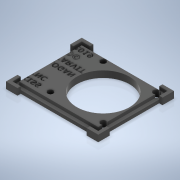
# Autodesk Inventor part: TNC Cover
Saved by Autodesk Inventor 2020.1 (Build 241239000, 239)
## iProperties
Created: 2019-09-18
Part Number: TNC Cover
Material: PC/ABS Plastic
Document SubType Name: Modeling
Designer: Logan
Density: 0.357273 g/cm^3
Appearance: Smooth - Black
Author: Logan
Autodesk Inventor part; units mm, degrees
(part 1 of 2)
ref_plane "YZ Plane" through (0, 0, 0) normal (1, 0, 0) x (0, 1, 0)
ref_plane "XZ Plane" through (0, 0, 0) normal (0, 1, 0) x (-1, 0, 0)
ref_plane "XY Plane" through (0, 0, 0) normal (0, 0, 1) x (1, 0, 0)
sketch "Sketch1" plane through (0, 0, 0) normal (0, 1, 0) x (-1, 0, 0)
  line L0 (0, 0) -> (52, 0)
  line L1 (52, 0) -> (52, -42)
  line L2 (52, -42) -> (0, -42)
  line L3 (0, -42) -> (0, 0)
  line L4 (52, 0) -> (0, 0)
  line L5 (0, 0) -> (0, -2)
  line L6 (0, -2) -> (52, -2)
  line L7 (52, -2) -> (52, 0)
  line L8 (0, 0) -> (2, 0)
  line L9 (2, 0) -> (2, -42)
  line L10 (2, -42) -> (0, -42)
  line L11 (0, -42) -> (0, 0)
  line L12 (52, -42) -> (0, -42)
  line L13 (0, -42) -> (0, -40)
  line L14 (0, -40) -> (52, -40)
  line L15 (52, -40) -> (52, -42)
  line L16 (52, -42) -> (50, -42)
  line L17 (50, -42) -> (50, 0)
  line L18 (50, 0) -> (52, 0)
  line L19 (52, 0) -> (52, -42)
  dimension "d0" = 52
  dimension "d1" = 42
  constraints: 40 end point, 10 parallel, 5 horizontal, 5 perpendicular, 4 point on line
  measures "d0" distance of L1.end L2.end
  measures "d1" distance of L0.end L1.end
extrude "Extrusion1" add sketch "Sketch1" along normal blind 2
sketch "Sketch2" plane through (0, 2, 0) normal (0, 1, 0) x (1, 0, 0)
  line L0 (-52, 42) -> (-52, 0) projected
  line L1 (0, 0) -> (0, 42) projected
  line L2 (-52, 0) -> (0, 0)
  line L3 (0, 0) -> (0, 2)
  line L4 (0, 2) -> (-52, 2)
  line L5 (-52, 2) -> (-52, 0)
  line L6 (0, 42) -> (-52, 42) projected
  line L7 (0, 0) -> (-2, 0)
  line L8 (-2, 0) -> (-2, 42)
  line L9 (-2, 42) -> (0, 42)
  line L10 (0, 42) -> (0, 0)
  line L11 (0, 42) -> (-52, 42)
  line L12 (-52, 42) -> (-52, 40)
  line L13 (-52, 40) -> (0, 40)
  line L14 (0, 40) -> (0, 42)
  line L15 (-52, 0) -> (0, 0) projected
  line L16 (-52, 42) -> (-50, 42)
  line L17 (-50, 42) -> (-50, 0)
  line L18 (-50, 0) -> (-52, 0)
  line L19 (-52, 0) -> (-52, 42)
  line L20 (-2, 2) -> (-50, 2)
  line L21 (-50, 2) -> (-50, 4)
  line L22 (-50, 4) -> (-2, 4)
  line L23 (-2, 4) -> (-2, 2)
  line L24 (-50, 2) -> (-48, 2)
  line L25 (-48, 2) -> (-48, 40)
  line L26 (-48, 40) -> (-50, 40)
  line L27 (-50, 40) -> (-50, 2)
  line L28 (-50, 40) -> (-2, 40)
  line L29 (-2, 40) -> (-2, 38)
  line L30 (-2, 38) -> (-50, 38)
  line L31 (-50, 38) -> (-50, 40)
  line L32 (-2, 40) -> (-4, 40)
  line L33 (-4, 40) -> (-4, 2)
  line L34 (-4, 2) -> (-2, 2)
  line L35 (-2, 2) -> (-2, 40)
  point P0 (-50, 2)
  point P1 (-2, 40)
  constraints: 64 end point, 16 parallel, 10 point on line, 8 horizontal, 8 perpendicular
extrude "Extrusion2" add sketch "Sketch2" along normal blind 2 contours L13 L25 L30 L17 | L17 L22 L25 L4 | L13 L33 L30 L25 | L30 L25 L22 L17 | L8 L30 L33 L13 | L25 L22 L33 L4 | L30 L33 L22 L25 | L8 L22 L33 L30 | L33 L22 L8 L4
sketch "Sketch3" plane through (0, 2, 0) normal (0, 1, 0) x (1, 0, 0)
  line L0 (-52, 0) -> (0, 0) projected
  line L1 (0, 0) -> (2, 0)
  line L2 (2, 0) -> (2, 5)
  line L3 (2, 5) -> (0, 5)
  line L4 (0, 5) -> (0, 0)
  line L5 (0, 0) -> (-5, 0)
  line L6 (-5, 0) -> (-5, -2)
  line L7 (-5, -2) -> (0, -2)
  line L8 (0, -2) -> (0, 0)
  line L9 (0, -2) -> (2, -2)
  line L10 (2, -2) -> (2, 0)
  line L11 (2, 0) -> (0, 0)
  line L12 (0, 0) -> (0, -2)
  line L13 (-52, 0) -> (-47, 0)
  line L14 (-47, 0) -> (-47, -2)
  line L15 (-47, -2) -> (-52, -2)
  line L16 (-52, -2) -> (-52, 0)
  line L17 (-52, -2) -> (-54, -2)
  line L18 (-54, -2) -> (-54, 0)
  line L19 (-54, 0) -> (-52, 0)
  line L20 (-52, 0) -> (-52, -2)
  line L21 (-52, 42) -> (-52, 0) projected
  line L22 (-54, 0) -> (-52, 0)
  line L23 (-52, 0) -> (-52, 5)
  line L24 (-52, 5) -> (-54, 5)
  line L25 (-54, 5) -> (-54, 0)
  line L26 (-52, 42) -> (-54, 42)
  line L27 (-54, 42) -> (-54, 37)
  line L28 (-54, 37) -> (-52, 37)
  line L29 (-52, 37) -> (-52, 42)
  line L30 (-54, 42) -> (-52, 42)
  line L31 (-52, 42) -> (-52, 44)
  line L32 (-52, 44) -> (-54, 44)
  line L33 (-54, 44) -> (-54, 42)
  line L34 (0, 42) -> (-52, 42) projected
  line L35 (-52, 44) -> (-47, 44)
  line L36 (-47, 44) -> (-47, 42)
  line L37 (-47, 42) -> (-52, 42)
  line L38 (-52, 42) -> (-52, 44)
  line L39 (0, 42) -> (-5, 42)
  line L40 (-5, 42) -> (-5, 44)
  line L41 (-5, 44) -> (0, 44)
  line L42 (0, 44) -> (0, 42)
  line L43 (0, 44) -> (2, 44)
  line L44 (2, 44) -> (2, 42)
  line L45 (2, 42) -> (0, 42)
  line L46 (0, 42) -> (0, 44)
  line L47 (0, 42) -> (2, 42)
  line L48 (2, 42) -> (2, 37)
  line L49 (2, 37) -> (0, 37)
  line L50 (0, 37) -> (0, 42)
  dimension "d6" = 5
  constraints: 96 end point, 24 parallel, 13 point on line, 12 horizontal, 12 perpendicular
  measures "d6" distance of L7.end L6.end
extrude "Extrusion3" add sketch "Sketch3" along normal mid plane 4
sketch "Sketch4" plane through (0, 0, 0) normal (0, -1, 0) x (1, 0, 0)
  line L0 (-52, -37) -> (-52, -42) projected
  line L1 (0, -5) -> (0, 0) projected
  line L2 (-52, -42) -> (0, -42)
  line L3 (0, -42) -> (0, 0)
  line L4 (0, 0) -> (-52, 0)
  line L5 (-52, 0) -> (-52, -42)
  line L6 (0, -5) -> (0, -37) projected
  line L7 (-52, -42) -> (0, -42)
  line L8 (0, -42) -> (0, -21)
  line L9 (0, -21) -> (-52, -21)
  line L10 (-52, -21) -> (-52, -42)
  line L11 (-52, -5) -> (-52, 0) projected
  line L12 (0, -21) -> (-52, -21)
  line L13 (-52, -21) -> (-52, 0)
  line L14 (-52, 0) -> (0, 0)
  line L15 (0, 0) -> (0, -21)
  line L16 (-52, -42) -> (-25, -42)
  line L17 (-25, -42) -> (-25, 0)
  line L18 (-25, 0) -> (-52, 0)
  line L19 (-52, 0) -> (-52, -42)
  line L20 (-51.6249, -4.1916) -> (-42.1937, -4.1916) construction
  line L21 (-42.1937, -4.1916) -> (-42.1937, -39.0347) construction
  line L22 (-42.1937, -39.0347) -> (-51.6249, -39.0347) construction
  line L23 (-51.6249, -39.0347) -> (-51.6249, -4.1916) construction
  line L24 (-3, -6) -> (-35, -6)
  line L25 (-35, -6) -> (-35, -38)
  line L26 (-35, -38) -> (-3, -38)
  line L27 (-3, -38) -> (-3, -6)
  circle A0 centre (-3, -6) radius 1.75
  circle A1 centre (-3, -38) radius 1.75
  circle A2 centre (-35, -38) radius 1.75
  circle A3 centre (-35, -6) radius 1.75
  line L28 (-35, -6) -> (-3, -6)
  line L29 (-3, -6) -> (1, -6)
  line L30 (-35, -6) -> (-39, -6)
  line L31 (-35, -6) -> (-35, -2)
  line L32 (-2, -2) -> (-50, -2) projected
  line L33 (-3, -6) -> (-3, -2)
  line L34 (-3, -38) -> (-3, -42)
  line L35 (0, -42) -> (-5, -42) projected
  line L36 (-3, -38) -> (1, -38)
  line L37 (1, -38) -> (-35, -38)
  line L38 (-35, -38) -> (-39, -38)
  line L39 (-39, -38) -> (-35, -38)
  line L40 (-35, -38) -> (-35, -42)
  line L41 (-39, -22) -> (-19, -22)
  circle A4 centre (-19, -22) radius 16
  line L42 (-48.5191, -7.4182) -> (-49.4824, -7.4182)
  line L43 (-49.4824, -7.4182) -> (-50.343, -6.1311)
  line L44 (-50.343, -6.1311) -> (-50.4997, -6.3469)
  line L45 (-50.4997, -6.3469) -> (-50.4997, -7.4182)
  line L46 (-50.4997, -7.4182) -> (-51.2961, -7.4182)
  line L47 (-51.2961, -7.4182) -> (-51.2961, -4.2482)
  line L48 (-51.2961, -4.2482) -> (-50.4997, -4.2482)
  line L49 (-50.4997, -4.2482) -> (-50.4997, -5.6636)
  line L50 (-50.4997, -5.6636) -> (-49.4824, -4.2482)
  line L51 (-49.4824, -4.2482) -> (-48.5654, -4.2482)
  line L52 (-48.5654, -4.2482) -> (-49.6957, -5.7201)
  line L53 (-49.6957, -5.7201) -> (-48.5191, -7.4182)
  line L54 (-46.6824, -7.4182) -> (-48.3881, -7.4182)
  line L55 (-48.3881, -7.4182) -> (-48.3881, -6.8658)
  line L56 (-48.3881, -6.8658) -> (-47.9334, -6.8658)
  line L57 (-47.9334, -6.8658) -> (-47.9334, -4.8005)
  line L58 (-47.9334, -4.8005) -> (-48.3881, -4.8005)
  line L59 (-48.3881, -4.8005) -> (-48.3881, -4.2482)
  line L60 (-48.3881, -4.2482) -> (-46.6824, -4.2482)
  line L61 (-46.6824, -4.2482) -> (-46.6824, -4.8005)
  line L62 (-46.6824, -4.8005) -> (-47.1371, -4.8005)
  line L63 (-47.1371, -4.8005) -> (-47.1371, -6.8658)
  line L64 (-47.1371, -6.8658) -> (-46.6824, -6.8658)
  line L65 (-46.6824, -6.8658) -> (-46.6824, -7.4182)
  spline S0 degree 2 poles (-45.1744, -7.4747) (-45.5392, -7.4747) (-46.089, -7.3334) (-46.3253, -7.2306) knots 0 0 0 1 2 2 2
  line L66 (-46.3253, -7.2306) -> (-46.3253, -6.4754)
  line L67 (-46.3253, -6.4754) -> (-46.2534, -6.4754)
  spline S1 degree 2 poles (-46.2534, -6.4754) (-46.0145, -6.6783) (-45.4416, -6.8967) (-45.1719, -6.8967) knots 0 0 0 1 2 2 2
  spline S2 degree 2 poles (-45.1719, -6.8967) (-45.1025, -6.8967) (-44.879, -6.8658) (-44.8122, -6.835) knots 0 0 0 1 2 2 2
  spline S3 degree 2 poles (-44.8122, -6.835) (-44.73, -6.7991) (-44.6144, -6.668) (-44.6144, -6.5627) knots 0 0 0 1 2 2 2
  spline S4 degree 2 poles (-44.6144, -6.5627) (-44.6144, -6.442) (-44.8019, -6.293) (-44.9304, -6.2596) knots 0 0 0 1 2 2 2
  spline S5 degree 2 poles (-44.9304, -6.2596) (-45.0922, -6.2159) (-45.4596, -6.1414) (-45.6214, -6.0849) knots 0 0 0 1 2 2 2
  spline S6 degree 2 poles (-45.6214, -6.0849) (-45.9888, -5.9565) (-46.3073, -5.5172) (-46.3073, -5.1884) knots 0 0 0 1 2 2 2
  spline S7 degree 2 poles (-46.3073, -5.1884) (-46.3073, -4.744) (-45.5546, -4.1916) (-44.9895, -4.1916) knots 0 0 0 1 2 2 2
  spline S8 degree 2 poles (-44.9895, -4.1916) (-44.7069, -4.1916) (-44.1469, -4.3072) (-43.926, -4.4049) knots 0 0 0 1 2 2 2
  line L68 (-43.926, -4.4049) -> (-43.926, -5.1293)
  line L69 (-43.926, -5.1293) -> (-43.9953, -5.1293)
  spline S9 degree 2 poles (-43.9953, -5.1293) (-44.1726, -4.9777) (-44.6812, -4.7696) (-44.9484, -4.7696) knots 0 0 0 1 2 2 2
  spline S10 degree 2 poles (-44.9484, -4.7696) (-45.0537, -4.7696) (-45.2181, -4.8005) (-45.3106, -4.8416) knots 0 0 0 1 2 2 2
  spline S11 degree 2 poles (-45.3106, -4.8416) (-45.3851, -4.875) (-45.493, -5.0085) (-45.493, -5.0908) knots 0 0 0 1 2 2 2
  spline S12 degree 2 poles (-45.493, -5.0908) (-45.493, -5.2141) (-45.3209, -5.3553) (-45.0742, -5.4119) knots 0 0 0 1 2 2 2
  spline S13 degree 2 poles (-45.0742, -5.4119) (-44.915, -5.4478) (-44.6196, -5.5172) (-44.45, -5.5763) knots 0 0 0 1 2 2 2
  spline S14 degree 2 poles (-44.45, -5.5763) (-44.1212, -5.697) (-43.8001, -6.0978) (-43.8001, -6.4266) knots 0 0 0 1 2 2 2
  spline S15 degree 2 poles (-43.8001, -6.4266) (-43.8001, -6.8992) (-44.5425, -7.4747) (-45.1744, -7.4747) knots 0 0 0 1 2 2 2
  spline S16 degree 2 poles (-42.4129, -7.4747) (-42.7777, -7.4747) (-43.3274, -7.3334) (-43.5637, -7.2306) knots 0 0 0 1 2 2 2
  line L70 (-43.5637, -7.2306) -> (-43.5637, -6.4754)
  line L71 (-43.5637, -6.4754) -> (-43.4918, -6.4754)
  spline S17 degree 2 poles (-43.4918, -6.4754) (-43.2529, -6.6783) (-42.68, -6.8967) (-42.4103, -6.8967) knots 0 0 0 1 2 2 2
  spline S18 degree 2 poles (-42.4103, -6.8967) (-42.341, -6.8967) (-42.1175, -6.8658) (-42.0507, -6.835) knots 0 0 0 1 2 2 2
  spline S19 degree 2 poles (-42.0507, -6.835) (-41.9685, -6.7991) (-41.8529, -6.668) (-41.8529, -6.5627) knots 0 0 0 1 2 2 2
  spline S20 degree 2 poles (-41.8529, -6.5627) (-41.8529, -6.442) (-42.0404, -6.293) (-42.1688, -6.2596) knots 0 0 0 1 2 2 2
  spline S21 degree 2 poles (-42.1688, -6.2596) (-42.3307, -6.2159) (-42.698, -6.1414) (-42.8599, -6.0849) knots 0 0 0 1 2 2 2
  spline S22 degree 2 poles (-42.8599, -6.0849) (-43.2272, -5.9565) (-43.5458, -5.5172) (-43.5458, -5.1884) knots 0 0 0 1 2 2 2
  spline S23 degree 2 poles (-43.5458, -5.1884) (-43.5458, -4.744) (-42.7931, -4.1916) (-42.2279, -4.1916) knots 0 0 0 1 2 2 2
  spline S24 degree 2 poles (-42.2279, -4.1916) (-41.9453, -4.1916) (-41.3853, -4.3072) (-41.1644, -4.4049) knots 0 0 0 1 2 2 2
  line L72 (-41.1644, -4.4049) -> (-41.1644, -5.1293)
  line L73 (-41.1644, -5.1293) -> (-41.2338, -5.1293)
  spline S25 degree 2 poles (-41.2338, -5.1293) (-41.411, -4.9777) (-41.9197, -4.7696) (-42.1868, -4.7696) knots 0 0 0 1 2 2 2
  spline S26 degree 2 poles (-42.1868, -4.7696) (-42.2921, -4.7696) (-42.4566, -4.8005) (-42.549, -4.8416) knots 0 0 0 1 2 2 2
  spline S27 degree 2 poles (-42.549, -4.8416) (-42.6235, -4.875) (-42.7314, -5.0085) (-42.7314, -5.0908) knots 0 0 0 1 2 2 2
  spline S28 degree 2 poles (-42.7314, -5.0908) (-42.7314, -5.2141) (-42.5593, -5.3553) (-42.3127, -5.4119) knots 0 0 0 1 2 2 2
  spline S29 degree 2 poles (-42.3127, -5.4119) (-42.1534, -5.4478) (-41.858, -5.5172) (-41.6885, -5.5763) knots 0 0 0 1 2 2 2
  spline S30 degree 2 poles (-41.6885, -5.5763) (-41.3596, -5.697) (-41.0385, -6.0978) (-41.0385, -6.4266) knots 0 0 0 1 2 2 2
  spline S31 degree 2 poles (-41.0385, -6.4266) (-41.0385, -6.8992) (-41.7809, -7.4747) (-42.4129, -7.4747) knots 0 0 0 1 2 2 2
  line L74 (-50.6873, -12.6375) -> (-50.6873, -10.0712)
  line L75 (-50.6873, -10.0712) -> (-51.6249, -10.0712)
  line L76 (-51.6249, -10.0712) -> (-51.6249, -9.4675)
  line L77 (-51.6249, -9.4675) -> (-48.9533, -9.4675)
  line L78 (-48.9533, -9.4675) -> (-48.9533, -10.0712)
  line L79 (-48.9533, -10.0712) -> (-49.8909, -10.0712)
  line L80 (-49.8909, -10.0712) -> (-49.8909, -12.6375)
  line L81 (-49.8909, -12.6375) -> (-50.6873, -12.6375)
  line L82 (-45.9117, -12.6375) -> (-46.6772, -12.6375)
  line L83 (-46.6772, -12.6375) -> (-47.9, -10.4282)
  line L84 (-47.9, -10.4282) -> (-47.9, -12.6375)
  line L85 (-47.9, -12.6375) -> (-48.627, -12.6375)
  line L86 (-48.627, -12.6375) -> (-48.627, -9.4675)
  line L87 (-48.627, -9.4675) -> (-47.6508, -9.4675)
  line L88 (-47.6508, -9.4675) -> (-46.6387, -11.2837)
  line L89 (-46.6387, -11.2837) -> (-46.6387, -9.4675)
  line L90 (-46.6387, -9.4675) -> (-45.9117, -9.4675)
  line L91 (-45.9117, -9.4675) -> (-45.9117, -12.6375)
  spline S32 degree 2 poles (-43.9003, -12.6991) (-44.6144, -12.6991) (-45.4519, -11.836) (-45.4519, -11.055) knots 0 0 0 1 2 2 2
  spline S33 degree 2 poles (-45.4519, -11.055) (-45.4519, -10.3024) (-44.6118, -9.4058) (-43.8977, -9.4058) knots 0 0 0 1 2 2 2
  spline S34 degree 2 poles (-43.8977, -9.4058) (-43.7102, -9.4058) (-43.407, -9.4495) (-43.2683, -9.4855) knots 0 0 0 1 2 2 2
  spline S35 degree 2 poles (-43.2683, -9.4855) (-43.1604, -9.5189) (-42.9061, -9.6293) (-42.8265, -9.6704) knots 0 0 0 1 2 2 2
  line L92 (-42.8265, -9.6704) -> (-42.8265, -10.4257)
  line L93 (-42.8265, -10.4257) -> (-42.9061, -10.4257)
  spline S36 degree 2 poles (-42.9061, -10.4257) (-42.9652, -10.3743) (-43.1399, -10.2304) (-43.2503, -10.1636) knots 0 0 0 1 2 2 2
  spline S37 degree 2 poles (-43.2503, -10.1636) (-43.3608, -10.0943) (-43.6254, -9.9992) (-43.7718, -9.9992) knots 0 0 0 1 2 2 2
  spline S38 degree 2 poles (-43.7718, -9.9992) (-43.9439, -9.9992) (-44.2291, -10.1071) (-44.3601, -10.2433) knots 0 0 0 1 2 2 2
  spline S39 degree 2 poles (-44.3601, -10.2433) (-44.4783, -10.364) (-44.6298, -10.7776) (-44.6298, -11.0576) knots 0 0 0 1 2 2 2
  spline S40 degree 2 poles (-44.6298, -11.0576) (-44.6298, -11.353) (-44.4731, -11.7564) (-44.3447, -11.8797) knots 0 0 0 1 2 2 2
  spline S41 degree 2 poles (-44.3447, -11.8797) (-44.2214, -12.0004) (-43.9182, -12.1057) (-43.7667, -12.1057) knots 0 0 0 1 2 2 2
  spline S42 degree 2 poles (-43.7667, -12.1057) (-43.61, -12.1057) (-43.3248, -12.0004) (-43.2272, -11.9362) knots 0 0 0 1 2 2 2
  spline S43 degree 2 poles (-43.2272, -11.9362) (-43.1193, -11.872) (-42.9575, -11.7358) (-42.8984, -11.6819) knots 0 0 0 1 2 2 2
  line L94 (-42.8984, -11.6819) -> (-42.8265, -11.6819)
  line L95 (-42.8265, -11.6819) -> (-42.8265, -12.4268)
  spline S44 degree 2 poles (-42.8265, -12.4268) (-42.9138, -12.4679) (-43.1424, -12.5707) (-43.2658, -12.6067) knots 0 0 0 1 2 2 2
  spline S45 degree 2 poles (-43.2658, -12.6067) (-43.4147, -12.6529) (-43.6742, -12.6991) (-43.9003, -12.6991) knots 0 0 0 1 2 2 2
  line L96 (-49.1819, -23.0761) -> (-51.2961, -23.0761)
  line L97 (-51.2961, -23.0761) -> (-51.2961, -19.9061)
  line L98 (-51.2961, -19.9061) -> (-50.4997, -19.9061)
  line L99 (-50.4997, -19.9061) -> (-50.4997, -22.4724)
  line L100 (-50.4997, -22.4724) -> (-49.1819, -22.4724)
  line L101 (-49.1819, -22.4724) -> (-49.1819, -23.0761)
  spline S46 degree 2 poles (-45.9168, -21.4911) (-45.9168, -22.2618) (-46.7389, -23.1429) (-47.453, -23.1429) knots 0 0 0 1 2 2 2
  spline S47 degree 2 poles (-47.453, -23.1429) (-48.1697, -23.1429) (-48.9867, -22.2515) (-48.9867, -21.4911) knots 0 0 0 1 2 2 2
  spline S48 degree 2 poles (-48.9867, -21.4911) (-48.9867, -20.7282) (-48.1697, -19.8393) (-47.453, -19.8393) knots 0 0 0 1 2 2 2
  spline S49 degree 2 poles (-47.453, -19.8393) (-46.7389, -19.8393) (-45.9168, -20.723) (-45.9168, -21.4911) knots 0 0 0 1 2 2 2
  spline S50 degree 2 poles (-46.7389, -21.4911) (-46.7389, -21.206) (-46.8545, -20.8078) (-46.9547, -20.6819) knots 0 0 0 1 2 2 2
  spline S51 degree 2 poles (-46.9547, -20.6819) (-47.0549, -20.5509) (-47.3117, -20.4379) (-47.4505, -20.4379) knots 0 0 0 1 2 2 2
  spline S52 degree 2 poles (-47.4505, -20.4379) (-47.5969, -20.4379) (-47.8358, -20.5432) (-47.9463, -20.6768) knots 0 0 0 1 2 2 2
  spline S53 degree 2 poles (-47.9463, -20.6768) (-48.0439, -20.8001) (-48.1646, -21.2085) (-48.1646, -21.4911) knots 0 0 0 1 2 2 2
  spline S54 degree 2 poles (-48.1646, -21.4911) (-48.1646, -21.784) (-48.049, -22.1693) (-47.9488, -22.3003) knots 0 0 0 1 2 2 2
  spline S55 degree 2 poles (-47.9488, -22.3003) (-47.8486, -22.4313) (-47.5892, -22.5444) (-47.4505, -22.5444) knots 0 0 0 1 2 2 2
  spline S56 degree 2 poles (-47.4505, -22.5444) (-47.3092, -22.5444) (-47.0471, -22.4236) (-46.9521, -22.2952) knots 0 0 0 1 2 2 2
  spline S57 degree 2 poles (-46.9521, -22.2952) (-46.8493, -22.1565) (-46.7389, -21.7891) (-46.7389, -21.4911) knots 0 0 0 1 2 2 2
  spline S58 degree 2 poles (-42.7982, -22.8963) (-43.0063, -22.9811) (-43.6716, -23.1429) (-43.9953, -23.1429) knots 0 0 0 1 2 2 2
  spline S59 degree 2 poles (-43.9953, -23.1429) (-44.7429, -23.1429) (-45.6291, -22.2798) (-45.6291, -21.4886) knots 0 0 0 1 2 2 2
  spline S60 degree 2 poles (-45.6291, -21.4886) (-45.6291, -20.7436) (-44.7429, -19.8445) (-43.9722, -19.8445) knots 0 0 0 1 2 2 2
  spline S61 degree 2 poles (-43.9722, -19.8445) (-43.574, -19.8445) (-43.0757, -19.996) (-42.8111, -20.1245) knots 0 0 0 1 2 2 2
  line L102 (-42.8111, -20.1245) -> (-42.8111, -20.8695)
  line L103 (-42.8111, -20.8695) -> (-42.883, -20.8695)
  spline S62 degree 2 poles (-42.883, -20.8695) (-42.9395, -20.8258) (-43.1553, -20.6588) (-43.258, -20.6023) knots 0 0 0 1 2 2 2
  spline S63 degree 2 poles (-43.258, -20.6023) (-43.3762, -20.5329) (-43.6896, -20.4353) (-43.8643, -20.4353) knots 0 0 0 1 2 2 2
  spline S64 degree 2 poles (-43.8643, -20.4353) (-44.0672, -20.4353) (-44.4038, -20.5638) (-44.5348, -20.6948) knots 0 0 0 1 2 2 2
  spline S65 degree 2 poles (-44.5348, -20.6948) (-44.6607, -20.8232) (-44.8071, -21.2163) (-44.8071, -21.4757) knots 0 0 0 1 2 2 2
  spline S66 degree 2 poles (-44.8071, -21.4757) (-44.8071, -22.0306) (-44.2496, -22.5598) (-43.7693, -22.5598) knots 0 0 0 1 2 2 2
  spline S67 degree 2 poles (-43.7693, -22.5598) (-43.7256, -22.5598) (-43.6126, -22.5546) (-43.5689, -22.5521) knots 0 0 0 1 2 2 2
  line L104 (-43.5689, -22.5521) -> (-43.5689, -21.9278)
  line L105 (-43.5689, -21.9278) -> (-44.1828, -21.9278)
  line L106 (-44.1828, -21.9278) -> (-44.1828, -21.3344)
  line L107 (-44.1828, -21.3344) -> (-42.7982, -21.3344)
  line L108 (-42.7982, -21.3344) -> (-42.7982, -22.8963)
  line L109 (-42.5388, -23.0761) -> (-41.4675, -19.9061)
  line L110 (-41.4675, -19.9061) -> (-40.5993, -19.9061)
  line L111 (-40.5993, -19.9061) -> (-39.528, -23.0761)
  line L112 (-39.528, -23.0761) -> (-40.3475, -23.0761)
  line L113 (-40.3475, -23.0761) -> (-40.5453, -22.4288)
  line L114 (-40.5453, -22.4288) -> (-41.542, -22.4288)
  line L115 (-41.542, -22.4288) -> (-41.7424, -23.0761)
  line L116 (-41.7424, -23.0761) -> (-42.5388, -23.0761)
  line L117 (-40.72, -21.8533) -> (-41.0437, -20.8052)
  line L118 (-41.0437, -20.8052) -> (-41.3699, -21.8533)
  line L119 (-41.3699, -21.8533) -> (-40.72, -21.8533)
  line L120 (-36.4968, -23.0761) -> (-37.2623, -23.0761)
  line L121 (-37.2623, -23.0761) -> (-38.4851, -20.8669)
  line L122 (-38.4851, -20.8669) -> (-38.4851, -23.0761)
  line L123 (-38.4851, -23.0761) -> (-39.2121, -23.0761)
  line L124 (-39.2121, -23.0761) -> (-39.2121, -19.9061)
  line L125 (-39.2121, -19.9061) -> (-38.2359, -19.9061)
  line L126 (-38.2359, -19.9061) -> (-37.2237, -21.7223)
  line L127 (-37.2237, -21.7223) -> (-37.2237, -19.9061)
  line L128 (-37.2237, -19.9061) -> (-36.4968, -19.9061)
  line L129 (-36.4968, -19.9061) -> (-36.4968, -23.0761)
  line L130 (-50.6873, -28.2954) -> (-50.6873, -25.7291)
  line L131 (-50.6873, -25.7291) -> (-51.6249, -25.7291)
  line L132 (-51.6249, -25.7291) -> (-51.6249, -25.1254)
  line L133 (-51.6249, -25.1254) -> (-48.9533, -25.1254)
  line L134 (-48.9533, -25.1254) -> (-48.9533, -25.7291)
  line L135 (-48.9533, -25.7291) -> (-49.8909, -25.7291)
  line L136 (-49.8909, -25.7291) -> (-49.8909, -28.2954)
  line L137 (-49.8909, -28.2954) -> (-50.6873, -28.2954)
  line L138 (-48.9687, -28.2954) -> (-47.8974, -25.1254)
  line L139 (-47.8974, -25.1254) -> (-47.0292, -25.1254)
  line L140 (-47.0292, -25.1254) -> (-45.9579, -28.2954)
  line L141 (-45.9579, -28.2954) -> (-46.7774, -28.2954)
  line L142 (-46.7774, -28.2954) -> (-46.9752, -27.6481)
  line L143 (-46.9752, -27.6481) -> (-47.9719, -27.6481)
  line L144 (-47.9719, -27.6481) -> (-48.1723, -28.2954)
  line L145 (-48.1723, -28.2954) -> (-48.9687, -28.2954)
  line L146 (-47.1499, -27.0727) -> (-47.4736, -26.0246)
  line L147 (-47.4736, -26.0246) -> (-47.7998, -27.0727)
  line L148 (-47.7998, -27.0727) -> (-47.1499, -27.0727)
  line L149 (-42.7134, -28.2954) -> (-43.6819, -28.2954)
  line L150 (-43.6819, -28.2954) -> (-44.563, -27.1317)
  line L151 (-44.563, -27.1317) -> (-44.8508, -27.1317)
  line L152 (-44.8508, -27.1317) -> (-44.8508, -28.2954)
  line L153 (-44.8508, -28.2954) -> (-45.642, -28.2954)
  line L154 (-45.642, -28.2954) -> (-45.642, -25.1254)
  line L155 (-45.642, -25.1254) -> (-44.3678, -25.1254)
  spline S68 degree 2 poles (-44.3678, -25.1254) (-44.1032, -25.1254) (-43.7127, -25.1922) (-43.5458, -25.295) knots 0 0 0 1 2 2 2
  spline S69 degree 2 poles (-43.5458, -25.295) (-43.3762, -25.4029) (-43.1758, -25.7394) (-43.1758, -25.9963) knots 0 0 0 1 2 2 2
  spline S70 degree 2 poles (-43.1758, -25.9963) (-43.1758, -26.3585) (-43.5047, -26.8132) (-43.7795, -26.9468) knots 0 0 0 1 2 2 2
  line L156 (-43.7795, -26.9468) -> (-42.7134, -28.2954)
  spline S71 degree 2 poles (-43.9927, -26.0965) (-43.9927, -25.9757) (-44.0852, -25.8036) (-44.1906, -25.7574) knots 0 0 0 1 2 2 2
  spline S72 degree 2 poles (-44.1906, -25.7574) (-44.265, -25.7266) (-44.4474, -25.7086) (-44.5836, -25.7086) knots 0 0 0 1 2 2 2
  line L157 (-44.5836, -25.7086) -> (-44.8508, -25.7086)
  line L158 (-44.8508, -25.7086) -> (-44.8508, -26.5615)
  line L159 (-44.8508, -26.5615) -> (-44.6221, -26.5615)
  spline S73 degree 2 poles (-44.6221, -26.5615) (-44.4577, -26.5615) (-44.2239, -26.5203) (-44.1443, -26.4561) knots 0 0 0 1 2 2 2
  spline S74 degree 2 poles (-44.1443, -26.4561) (-44.0672, -26.3945) (-43.9927, -26.2301) (-43.9927, -26.0965) knots 0 0 0 1 2 2 2
  line L160 (-39.8312, -25.1254) -> (-40.9204, -28.2954)
  line L161 (-40.9204, -28.2954) -> (-41.7501, -28.2954)
  line L162 (-41.7501, -28.2954) -> (-42.8393, -25.1254)
  line L163 (-42.8393, -25.1254) -> (-42.0147, -25.1254)
  line L164 (-42.0147, -25.1254) -> (-41.3237, -27.2756)
  line L165 (-41.3237, -27.2756) -> (-40.6352, -25.1254)
  line L166 (-40.6352, -25.1254) -> (-39.8312, -25.1254)
  line L167 (-37.9584, -28.2954) -> (-39.6642, -28.2954)
  line L168 (-39.6642, -28.2954) -> (-39.6642, -27.7431)
  line L169 (-39.6642, -27.7431) -> (-39.2095, -27.7431)
  line L170 (-39.2095, -27.7431) -> (-39.2095, -25.6778)
  line L171 (-39.2095, -25.6778) -> (-39.6642, -25.6778)
  line L172 (-39.6642, -25.6778) -> (-39.6642, -25.1254)
  line L173 (-39.6642, -25.1254) -> (-37.9584, -25.1254)
  line L174 (-37.9584, -25.1254) -> (-37.9584, -25.6778)
  line L175 (-37.9584, -25.6778) -> (-38.4131, -25.6778)
  line L176 (-38.4131, -25.6778) -> (-38.4131, -27.7431)
  line L177 (-38.4131, -27.7431) -> (-37.9584, -27.7431)
  line L178 (-37.9584, -27.7431) -> (-37.9584, -28.2954)
  line L179 (-36.8204, -28.2954) -> (-36.8204, -25.7291)
  line L180 (-36.8204, -25.7291) -> (-37.7581, -25.7291)
  line L181 (-37.7581, -25.7291) -> (-37.7581, -25.1254)
  line L182 (-37.7581, -25.1254) -> (-35.0864, -25.1254)
  line L183 (-35.0864, -25.1254) -> (-35.0864, -25.7291)
  line L184 (-35.0864, -25.7291) -> (-36.0241, -25.7291)
  line L185 (-36.0241, -25.7291) -> (-36.0241, -28.2954)
  line L186 (-36.0241, -28.2954) -> (-36.8204, -28.2954)
  spline S75 degree 2 poles (-47.7587, -32.1199) (-47.7587, -32.8828) (-48.8377, -33.9618) (-49.6006, -33.9618) knots 0 0 0 1 2 2 2
  spline S76 degree 2 poles (-49.6006, -33.9618) (-50.3636, -33.9618) (-51.4425, -32.8828) (-51.4425, -32.1199) knots 0 0 0 1 2 2 2
  spline S77 degree 2 poles (-51.4425, -32.1199) (-51.4425, -31.3569) (-50.3636, -30.278) (-49.6006, -30.278) knots 0 0 0 1 2 2 2
  spline S78 degree 2 poles (-49.6006, -30.278) (-48.8377, -30.278) (-47.7587, -31.3569) (-47.7587, -32.1199) knots 0 0 0 1 2 2 2
  spline S79 degree 2 poles (-48.1646, -32.1199) (-48.1646, -31.5265) (-49.0072, -30.6736) (-49.6006, -30.6736) knots 0 0 0 1 2 2 2
  spline S80 degree 2 poles (-49.6006, -30.6736) (-50.194, -30.6736) (-51.0366, -31.5265) (-51.0366, -32.1199) knots 0 0 0 1 2 2 2
  spline S81 degree 2 poles (-51.0366, -32.1199) (-51.0366, -32.7133) (-50.194, -33.5661) (-49.6006, -33.5661) knots 0 0 0 1 2 2 2
  spline S82 degree 2 poles (-49.6006, -33.5661) (-49.0072, -33.5661) (-48.1646, -32.7133) (-48.1646, -32.1199) knots 0 0 0 1 2 2 2
  spline S83 degree 2 poles (-48.925, -32.9239) (-48.9815, -32.9496) (-49.1023, -33.0036) (-49.187, -33.0267) knots 0 0 0 1 2 2 2
  spline S84 degree 2 poles (-49.187, -33.0267) (-49.2744, -33.0524) (-49.4105, -33.0781) (-49.5158, -33.0781) knots 0 0 0 1 2 2 2
  spline S85 degree 2 poles (-49.5158, -33.0781) (-49.7136, -33.0781) (-50.0707, -32.9599) (-50.2017, -32.8392) knots 0 0 0 1 2 2 2
  spline S86 degree 2 poles (-50.2017, -32.8392) (-50.3353, -32.7158) (-50.4894, -32.3588) (-50.4894, -32.1096) knots 0 0 0 1 2 2 2
  spline S87 degree 2 poles (-50.4894, -32.1096) (-50.4894, -31.8733) (-50.3379, -31.5136) (-50.2043, -31.3877) knots 0 0 0 1 2 2 2
  spline S88 degree 2 poles (-50.2043, -31.3877) (-50.0733, -31.2644) (-49.7136, -31.1334) (-49.5158, -31.1334) knots 0 0 0 1 2 2 2
  spline S89 degree 2 poles (-49.5158, -31.1334) (-49.354, -31.1334) (-49.0534, -31.2208) (-48.925, -31.285) knots 0 0 0 1 2 2 2
  line L187 (-48.925, -31.285) -> (-48.925, -31.7191)
  line L188 (-48.925, -31.7191) -> (-48.9687, -31.7191)
  spline S90 degree 2 poles (-48.9687, -31.7191) (-49.0098, -31.6883) (-49.1048, -31.6215) (-49.1819, -31.583) knots 0 0 0 1 2 2 2
  spline S91 degree 2 poles (-49.1819, -31.583) (-49.2487, -31.5496) (-49.4182, -31.5033) (-49.5056, -31.5033) knots 0 0 0 1 2 2 2
  spline S92 degree 2 poles (-49.5056, -31.5033) (-49.7316, -31.5033) (-49.9757, -31.8116) (-49.9757, -32.1096) knots 0 0 0 1 2 2 2
  spline S93 degree 2 poles (-49.9757, -32.1096) (-49.9757, -32.3999) (-49.7265, -32.7081) (-49.5056, -32.7081) knots 0 0 0 1 2 2 2
  spline S94 degree 2 poles (-49.5056, -32.7081) (-49.4079, -32.7081) (-49.2333, -32.6593) (-49.1716, -32.6259) knots 0 0 0 1 2 2 2
  spline S95 degree 2 poles (-49.1716, -32.6259) (-49.0997, -32.5874) (-49.0021, -32.5206) (-48.9687, -32.4924) knots 0 0 0 1 2 2 2
  line L189 (-48.9687, -32.4924) -> (-48.925, -32.4924)
  line L190 (-48.925, -32.4924) -> (-48.925, -32.9239)
  spline S96 degree 2 poles (-43.7102, -32.1199) (-43.7102, -32.8828) (-44.7891, -33.9618) (-45.5521, -33.9618) knots 0 0 0 1 2 2 2
  spline S97 degree 2 poles (-45.5521, -33.9618) (-46.315, -33.9618) (-47.3939, -32.8828) (-47.3939, -32.1199) knots 0 0 0 1 2 2 2
  spline S98 degree 2 poles (-47.3939, -32.1199) (-47.3939, -31.3569) (-46.315, -30.278) (-45.5521, -30.278) knots 0 0 0 1 2 2 2
  spline S99 degree 2 poles (-45.5521, -30.278) (-44.7891, -30.278) (-43.7102, -31.3569) (-43.7102, -32.1199) knots 0 0 0 1 2 2 2
  spline S100 degree 2 poles (-44.1161, -32.1199) (-44.1161, -31.5265) (-44.9586, -30.6736) (-45.5521, -30.6736) knots 0 0 0 1 2 2 2
  spline S101 degree 2 poles (-45.5521, -30.6736) (-46.1455, -30.6736) (-46.9881, -31.5265) (-46.9881, -32.1199) knots 0 0 0 1 2 2 2
  spline S102 degree 2 poles (-46.9881, -32.1199) (-46.9881, -32.7133) (-46.1455, -33.5661) (-45.5521, -33.5661) knots 0 0 0 1 2 2 2
  spline S103 degree 2 poles (-45.5521, -33.5661) (-44.9586, -33.5661) (-44.1161, -32.7133) (-44.1161, -32.1199) knots 0 0 0 1 2 2 2
  spline S104 degree 2 poles (-44.8764, -32.9239) (-44.933, -32.9496) (-45.0537, -33.0036) (-45.1385, -33.0267) knots 0 0 0 1 2 2 2
  spline S105 degree 2 poles (-45.1385, -33.0267) (-45.2258, -33.0524) (-45.362, -33.0781) (-45.4673, -33.0781) knots 0 0 0 1 2 2 2
  spline S106 degree 2 poles (-45.4673, -33.0781) (-45.6651, -33.0781) (-46.0222, -32.9599) (-46.1532, -32.8392) knots 0 0 0 1 2 2 2
  spline S107 degree 2 poles (-46.1532, -32.8392) (-46.2868, -32.7158) (-46.4409, -32.3588) (-46.4409, -32.1096) knots 0 0 0 1 2 2 2
  spline S108 degree 2 poles (-46.4409, -32.1096) (-46.4409, -31.8733) (-46.2893, -31.5136) (-46.1557, -31.3877) knots 0 0 0 1 2 2 2
  spline S109 degree 2 poles (-46.1557, -31.3877) (-46.0247, -31.2644) (-45.6651, -31.1334) (-45.4673, -31.1334) knots 0 0 0 1 2 2 2
  spline S110 degree 2 poles (-45.4673, -31.1334) (-45.3054, -31.1334) (-45.0049, -31.2208) (-44.8764, -31.285) knots 0 0 0 1 2 2 2
  line L191 (-44.8764, -31.285) -> (-44.8764, -31.7191)
  line L192 (-44.8764, -31.7191) -> (-44.9201, -31.7191)
  spline S111 degree 2 poles (-44.9201, -31.7191) (-44.9612, -31.6883) (-45.0563, -31.6215) (-45.1333, -31.583) knots 0 0 0 1 2 2 2
  spline S112 degree 2 poles (-45.1333, -31.583) (-45.2001, -31.5496) (-45.3697, -31.5033) (-45.457, -31.5033) knots 0 0 0 1 2 2 2
  spline S113 degree 2 poles (-45.457, -31.5033) (-45.6831, -31.5033) (-45.9271, -31.8116) (-45.9271, -32.1096) knots 0 0 0 1 2 2 2
  spline S114 degree 2 poles (-45.9271, -32.1096) (-45.9271, -32.3999) (-45.6779, -32.7081) (-45.457, -32.7081) knots 0 0 0 1 2 2 2
  spline S115 degree 2 poles (-45.457, -32.7081) (-45.3594, -32.7081) (-45.1847, -32.6593) (-45.1231, -32.6259) knots 0 0 0 1 2 2 2
  spline S116 degree 2 poles (-45.1231, -32.6259) (-45.0511, -32.5874) (-44.9535, -32.5206) (-44.9201, -32.4924) knots 0 0 0 1 2 2 2
  line L193 (-44.9201, -32.4924) -> (-44.8764, -32.4924)
  line L194 (-44.8764, -32.4924) -> (-44.8764, -32.9239)
  line L195 (-48.9738, -38.7341) -> (-51.3038, -38.7341)
  line L196 (-51.3038, -38.7341) -> (-51.3038, -38.2177)
  spline S117 degree 2 poles (-51.3038, -38.2177) (-51.0084, -37.9814) (-50.5357, -37.5652) (-50.3584, -37.3777) knots 0 0 0 1 2 2 2
  spline S118 degree 2 poles (-50.3584, -37.3777) (-50.1247, -37.1337) (-49.9166, -36.7612) (-49.9166, -36.566) knots 0 0 0 1 2 2 2
  spline S119 degree 2 poles (-49.9166, -36.566) (-49.9166, -36.345) (-50.1812, -36.1087) (-50.4175, -36.1087) knots 0 0 0 1 2 2 2
  spline S120 degree 2 poles (-50.4175, -36.1087) (-50.5383, -36.1087) (-50.754, -36.1678) (-50.8645, -36.214) knots 0 0 0 1 2 2 2
  spline S121 degree 2 poles (-50.8645, -36.214) (-50.9724, -36.2628) (-51.1265, -36.3656) (-51.1651, -36.3913) knots 0 0 0 1 2 2 2
  line L197 (-51.1651, -36.3913) -> (-51.2267, -36.3913)
  line L198 (-51.2267, -36.3913) -> (-51.2267, -35.7002)
  spline S122 degree 2 poles (-51.2267, -35.7002) (-51.0931, -35.636) (-50.5228, -35.5024) (-50.2582, -35.5024) knots 0 0 0 1 2 2 2
  spline S123 degree 2 poles (-50.2582, -35.5024) (-49.6931, -35.5024) (-49.1125, -36.0059) (-49.1125, -36.4606) knots 0 0 0 1 2 2 2
  spline S124 degree 2 poles (-49.1125, -36.4606) (-49.1125, -36.7406) (-49.3771, -37.2801) (-49.6828, -37.5884) knots 0 0 0 1 2 2 2
  spline S125 degree 2 poles (-49.6828, -37.5884) (-49.8755, -37.7785) (-50.2377, -38.0739) (-50.3173, -38.1355) knots 0 0 0 1 2 2 2
  line L199 (-50.3173, -38.1355) -> (-48.9738, -38.1355)
  line L200 (-48.9738, -38.1355) -> (-48.9738, -38.7341)
  spline S126 degree 2 poles (-46.2379, -37.1491) (-46.2379, -37.5601) (-46.369, -38.1766) (-46.5154, -38.3847) knots 0 0 0 1 2 2 2
  spline S127 degree 2 poles (-46.5154, -38.3847) (-46.6592, -38.5902) (-47.1242, -38.8009) (-47.4582, -38.8009) knots 0 0 0 1 2 2 2
  spline S128 degree 2 poles (-47.4582, -38.8009) (-47.7947, -38.8009) (-48.2571, -38.5902) (-48.4035, -38.3796) knots 0 0 0 1 2 2 2
  spline S129 degree 2 poles (-48.4035, -38.3796) (-48.5499, -38.1715) (-48.681, -37.5601) (-48.681, -37.1491) knots 0 0 0 1 2 2 2
  spline S130 degree 2 poles (-48.681, -37.1491) (-48.681, -36.7278) (-48.5499, -36.1318) (-48.4009, -35.916) knots 0 0 0 1 2 2 2
  spline S131 degree 2 poles (-48.4009, -35.916) (-48.252, -35.7054) (-47.7818, -35.4999) (-47.4582, -35.4999) knots 0 0 0 1 2 2 2
  spline S132 degree 2 poles (-47.4582, -35.4999) (-47.1165, -35.4999) (-46.6592, -35.7157) (-46.5128, -35.9289) knots 0 0 0 1 2 2 2
  spline S133 degree 2 poles (-46.5128, -35.9289) (-46.369, -36.1369) (-46.2379, -36.7509) (-46.2379, -37.1491) knots 0 0 0 1 2 2 2
  spline S134 degree 2 poles (-47.0369, -37.1491) (-47.0369, -36.5608) (-47.2295, -36.0856) (-47.4582, -36.0856) knots 0 0 0 1 2 2 2
  spline S135 degree 2 poles (-47.4582, -36.0856) (-47.6868, -36.0856) (-47.882, -36.5608) (-47.882, -37.1517) knots 0 0 0 1 2 2 2
  spline S136 degree 2 poles (-47.882, -37.1517) (-47.882, -37.7322) (-47.6868, -38.2152) (-47.4582, -38.2152) knots 0 0 0 1 2 2 2
  spline S137 degree 2 poles (-47.4582, -38.2152) (-47.2321, -38.2152) (-47.0369, -37.7322) (-47.0369, -37.1491) knots 0 0 0 1 2 2 2
  line L201 (-43.5612, -38.7341) -> (-45.6548, -38.7341)
  line L202 (-45.6548, -38.7341) -> (-45.6548, -38.1818)
  line L203 (-45.6548, -38.1818) -> (-44.9869, -38.1818)
  line L204 (-44.9869, -38.1818) -> (-44.9869, -36.5043)
  line L205 (-44.9869, -36.5043) -> (-45.6548, -36.5043)
  line L206 (-45.6548, -36.5043) -> (-45.6548, -35.988)
  spline S138 degree 2 poles (-45.6548, -35.988) (-45.5084, -35.988) (-45.2181, -35.9494) (-45.1308, -35.9083) knots 0 0 0 1 2 2 2
  spline S139 degree 2 poles (-45.1308, -35.9083) (-45.0306, -35.8569) (-44.9175, -35.6848) (-44.9073, -35.5564) knots 0 0 0 1 2 2 2
  line L207 (-44.9073, -35.5564) -> (-44.2137, -35.5564)
  line L208 (-44.2137, -35.5564) -> (-44.2137, -38.1818)
  line L209 (-44.2137, -38.1818) -> (-43.5612, -38.1818)
  line L210 (-43.5612, -38.1818) -> (-43.5612, -38.7341)
  spline S140 degree 2 poles (-40.7251, -36.9718) (-40.7251, -37.3752) (-40.9127, -38.0482) (-41.1105, -38.2897) knots 0 0 0 1 2 2 2
  spline S141 degree 2 poles (-41.1105, -38.2897) (-41.316, -38.5337) (-41.9222, -38.7957) (-42.3641, -38.7957) knots 0 0 0 1 2 2 2
  spline S142 degree 2 poles (-42.3641, -38.7957) (-42.5131, -38.7957) (-42.8368, -38.7572) (-42.8907, -38.7418) knots 0 0 0 1 2 2 2
  line L211 (-42.8907, -38.7418) -> (-42.8907, -38.1201)
  line L212 (-42.8907, -38.1201) -> (-42.829, -38.1201)
  spline S143 degree 2 poles (-42.829, -38.1201) (-42.77, -38.151) (-42.549, -38.2177) (-42.3564, -38.2177) knots 0 0 0 1 2 2 2
  spline S144 degree 2 poles (-42.3564, -38.2177) (-42.1997, -38.2177) (-41.9094, -38.1355) (-41.8066, -38.0456) knots 0 0 0 1 2 2 2
  spline S145 degree 2 poles (-41.8066, -38.0456) (-41.6962, -37.9506) (-41.5523, -37.6706) (-41.5266, -37.4599) knots 0 0 0 1 2 2 2
  spline S146 degree 2 poles (-41.5266, -37.4599) (-41.6962, -37.5652) (-41.989, -37.6783) (-42.2074, -37.6783) knots 0 0 0 1 2 2 2
  spline S147 degree 2 poles (-42.2074, -37.6783) (-42.3692, -37.6783) (-42.6698, -37.5909) (-42.7931, -37.4985) knots 0 0 0 1 2 2 2
  spline S148 degree 2 poles (-42.7931, -37.4985) (-42.9575, -37.3726) (-43.1502, -36.9693) (-43.1502, -36.6507) knots 0 0 0 1 2 2 2
  spline S149 degree 2 poles (-43.1502, -36.6507) (-43.1502, -36.4015) (-42.9806, -35.9828) (-42.8265, -35.8287) knots 0 0 0 1 2 2 2
  spline S150 degree 2 poles (-42.8265, -35.8287) (-42.6723, -35.6746) (-42.2254, -35.4999) (-41.9505, -35.4999) knots 0 0 0 1 2 2 2
  spline S151 degree 2 poles (-41.9505, -35.4999) (-41.673, -35.4999) (-41.244, -35.654) (-41.0899, -35.8158) knots 0 0 0 1 2 2 2
  spline S152 degree 2 poles (-41.0899, -35.8158) (-40.9101, -35.9957) (-40.7251, -36.566) (-40.7251, -36.9718) knots 0 0 0 1 2 2 2
  spline S153 degree 2 poles (-41.5138, -36.8537) (-41.5138, -36.5942) (-41.6011, -36.2603) (-41.6808, -36.1678) knots 0 0 0 1 2 2 2
  spline S154 degree 2 poles (-41.6808, -36.1678) (-41.7347, -36.0984) (-41.8734, -36.0393) (-41.9531, -36.0393) knots 0 0 0 1 2 2 2
  spline S155 degree 2 poles (-41.9531, -36.0393) (-42.025, -36.0393) (-42.1586, -36.0958) (-42.2202, -36.1678) knots 0 0 0 1 2 2 2
  spline S156 degree 2 poles (-42.2202, -36.1678) (-42.2742, -36.2294) (-42.3512, -36.4683) (-42.3512, -36.6096) knots 0 0 0 1 2 2 2
  spline S157 degree 2 poles (-42.3512, -36.6096) (-42.3512, -36.7638) (-42.2716, -36.9616) (-42.2048, -37.0206) knots 0 0 0 1 2 2 2
  spline S158 degree 2 poles (-42.2048, -37.0206) (-42.1354, -37.0797) (-41.9633, -37.126) (-41.8554, -37.126) knots 0 0 0 1 2 2 2
  spline S159 degree 2 poles (-41.8554, -37.126) (-41.7655, -37.126) (-41.578, -37.0772) (-41.5189, -37.0515) knots 0 0 0 1 2 2 2
  spline S160 degree 2 poles (-41.5189, -37.0515) (-41.5189, -37.0284) (-41.5138, -36.941) (-41.5138, -36.8537) knots 0 0 0 1 2 2 2
  line L213 (-48.5191, -7.4182) -> (-49.4824, -7.4182)
  line L214 (-49.4824, -7.4182) -> (-50.343, -6.1311)
  line L215 (-50.343, -6.1311) -> (-50.4997, -6.3469)
  line L216 (-50.4997, -6.3469) -> (-50.4997, -7.4182)
  line L217 (-50.4997, -7.4182) -> (-51.2961, -7.4182)
  line L218 (-51.2961, -7.4182) -> (-51.2961, -4.2482)
  line L219 (-51.2961, -4.2482) -> (-50.4997, -4.2482)
  line L220 (-50.4997, -4.2482) -> (-50.4997, -5.6636)
  line L221 (-50.4997, -5.6636) -> (-49.4824, -4.2482)
  line L222 (-49.4824, -4.2482) -> (-48.5654, -4.2482)
  line L223 (-48.5654, -4.2482) -> (-49.6957, -5.7201)
  line L224 (-49.6957, -5.7201) -> (-48.5191, -7.4182)
  line L225 (-46.6824, -7.4182) -> (-48.3881, -7.4182)
  line L226 (-48.3881, -7.4182) -> (-48.3881, -6.8658)
  line L227 (-48.3881, -6.8658) -> (-47.9334, -6.8658)
  line L228 (-47.9334, -6.8658) -> (-47.9334, -4.8005)
  line L229 (-47.9334, -4.8005) -> (-48.3881, -4.8005)
  line L230 (-48.3881, -4.8005) -> (-48.3881, -4.2482)
  line L231 (-48.3881, -4.2482) -> (-46.6824, -4.2482)
  line L232 (-46.6824, -4.2482) -> (-46.6824, -4.8005)
  line L233 (-46.6824, -4.8005) -> (-47.1371, -4.8005)
  line L234 (-47.1371, -4.8005) -> (-47.1371, -6.8658)
  line L235 (-47.1371, -6.8658) -> (-46.6824, -6.8658)
  line L236 (-46.6824, -6.8658) -> (-46.6824, -7.4182)
  spline S161 degree 2 poles (-45.1744, -7.4747) (-45.5392, -7.4747) (-46.089, -7.3334) (-46.3253, -7.2306) knots 0 0 0 1 2 2 2
  line L237 (-46.3253, -7.2306) -> (-46.3253, -6.4754)
  line L238 (-46.3253, -6.4754) -> (-46.2534, -6.4754)
  spline S162 degree 2 poles (-46.2534, -6.4754) (-46.0145, -6.6783) (-45.4416, -6.8967) (-45.1719, -6.8967) knots 0 0 0 1 2 2 2
  spline S163 degree 2 poles (-45.1719, -6.8967) (-45.1025, -6.8967) (-44.879, -6.8658) (-44.8122, -6.835) knots 0 0 0 1 2 2 2
  spline S164 degree 2 poles (-44.8122, -6.835) (-44.73, -6.7991) (-44.6144, -6.668) (-44.6144, -6.5627) knots 0 0 0 1 2 2 2
  spline S165 degree 2 poles (-44.6144, -6.5627) (-44.6144, -6.442) (-44.8019, -6.293) (-44.9304, -6.2596) knots 0 0 0 1 2 2 2
  spline S166 degree 2 poles (-44.9304, -6.2596) (-45.0922, -6.2159) (-45.4596, -6.1414) (-45.6214, -6.0849) knots 0 0 0 1 2 2 2
  spline S167 degree 2 poles (-45.6214, -6.0849) (-45.9888, -5.9565) (-46.3073, -5.5172) (-46.3073, -5.1884) knots 0 0 0 1 2 2 2
  spline S168 degree 2 poles (-46.3073, -5.1884) (-46.3073, -4.744) (-45.5546, -4.1916) (-44.9895, -4.1916) knots 0 0 0 1 2 2 2
  spline S169 degree 2 poles (-44.9895, -4.1916) (-44.7069, -4.1916) (-44.1469, -4.3072) (-43.926, -4.4049) knots 0 0 0 1 2 2 2
  line L239 (-43.926, -4.4049) -> (-43.926, -5.1293)
  line L240 (-43.926, -5.1293) -> (-43.9953, -5.1293)
  spline S170 degree 2 poles (-43.9953, -5.1293) (-44.1726, -4.9777) (-44.6812, -4.7696) (-44.9484, -4.7696) knots 0 0 0 1 2 2 2
  spline S171 degree 2 poles (-44.9484, -4.7696) (-45.0537, -4.7696) (-45.2181, -4.8005) (-45.3106, -4.8416) knots 0 0 0 1 2 2 2
  spline S172 degree 2 poles (-45.3106, -4.8416) (-45.3851, -4.875) (-45.493, -5.0085) (-45.493, -5.0908) knots 0 0 0 1 2 2 2
  spline S173 degree 2 poles (-45.493, -5.0908) (-45.493, -5.2141) (-45.3209, -5.3553) (-45.0742, -5.4119) knots 0 0 0 1 2 2 2
  spline S174 degree 2 poles (-45.0742, -5.4119) (-44.915, -5.4478) (-44.6196, -5.5172) (-44.45, -5.5763) knots 0 0 0 1 2 2 2
  spline S175 degree 2 poles (-44.45, -5.5763) (-44.1212, -5.697) (-43.8001, -6.0978) (-43.8001, -6.4266) knots 0 0 0 1 2 2 2
  spline S176 degree 2 poles (-43.8001, -6.4266) (-43.8001, -6.8992) (-44.5425, -7.4747) (-45.1744, -7.4747) knots 0 0 0 1 2 2 2
  spline S177 degree 2 poles (-42.4129, -7.4747) (-42.7777, -7.4747) (-43.3274, -7.3334) (-43.5637, -7.2306) knots 0 0 0 1 2 2 2
  line L241 (-43.5637, -7.2306) -> (-43.5637, -6.4754)
  line L242 (-43.5637, -6.4754) -> (-43.4918, -6.4754)
  spline S178 degree 2 poles (-43.4918, -6.4754) (-43.2529, -6.6783) (-42.68, -6.8967) (-42.4103, -6.8967) knots 0 0 0 1 2 2 2
  spline S179 degree 2 poles (-42.4103, -6.8967) (-42.341, -6.8967) (-42.1175, -6.8658) (-42.0507, -6.835) knots 0 0 0 1 2 2 2
  spline S180 degree 2 poles (-42.0507, -6.835) (-41.9685, -6.7991) (-41.8529, -6.668) (-41.8529, -6.5627) knots 0 0 0 1 2 2 2
  spline S181 degree 2 poles (-41.8529, -6.5627) (-41.8529, -6.442) (-42.0404, -6.293) (-42.1688, -6.2596) knots 0 0 0 1 2 2 2
  spline S182 degree 2 poles (-42.1688, -6.2596) (-42.3307, -6.2159) (-42.698, -6.1414) (-42.8599, -6.0849) knots 0 0 0 1 2 2 2
  spline S183 degree 2 poles (-42.8599, -6.0849) (-43.2272, -5.9565) (-43.5458, -5.5172) (-43.5458, -5.1884) knots 0 0 0 1 2 2 2
  spline S184 degree 2 poles (-43.5458, -5.1884) (-43.5458, -4.744) (-42.7931, -4.1916) (-42.2279, -4.1916) knots 0 0 0 1 2 2 2
  spline S185 degree 2 poles (-42.2279, -4.1916) (-41.9453, -4.1916) (-41.3853, -4.3072) (-41.1644, -4.4049) knots 0 0 0 1 2 2 2
  line L243 (-41.1644, -4.4049) -> (-41.1644, -5.1293)
  line L244 (-41.1644, -5.1293) -> (-41.2338, -5.1293)
  spline S186 degree 2 poles (-41.2338, -5.1293) (-41.411, -4.9777) (-41.9197, -4.7696) (-42.1868, -4.7696) knots 0 0 0 1 2 2 2
  spline S187 degree 2 poles (-42.1868, -4.7696) (-42.2921, -4.7696) (-42.4566, -4.8005) (-42.549, -4.8416) knots 0 0 0 1 2 2 2
  spline S188 degree 2 poles (-42.549, -4.8416) (-42.6235, -4.875) (-42.7314, -5.0085) (-42.7314, -5.0908) knots 0 0 0 1 2 2 2
  spline S189 degree 2 poles (-42.7314, -5.0908) (-42.7314, -5.2141) (-42.5593, -5.3553) (-42.3127, -5.4119) knots 0 0 0 1 2 2 2
  spline S190 degree 2 poles (-42.3127, -5.4119) (-42.1534, -5.4478) (-41.858, -5.5172) (-41.6885, -5.5763) knots 0 0 0 1 2 2 2
  spline S191 degree 2 poles (-41.6885, -5.5763) (-41.3596, -5.697) (-41.0385, -6.0978) (-41.0385, -6.4266) knots 0 0 0 1 2 2 2
  spline S192 degree 2 poles (-41.0385, -6.4266) (-41.0385, -6.8992) (-41.7809, -7.4747) (-42.4129, -7.4747) knots 0 0 0 1 2 2 2
  line L245 (-50.6873, -12.6375) -> (-50.6873, -10.0712)
  line L246 (-50.6873, -10.0712) -> (-51.6249, -10.0712)
  line L247 (-51.6249, -10.0712) -> (-51.6249, -9.4675)
  line L248 (-51.6249, -9.4675) -> (-48.9533, -9.4675)
  line L249 (-48.9533, -9.4675) -> (-48.9533, -10.0712)
  line L250 (-48.9533, -10.0712) -> (-49.8909, -10.0712)
  line L251 (-49.8909, -10.0712) -> (-49.8909, -12.6375)
  line L252 (-49.8909, -12.6375) -> (-50.6873, -12.6375)
  line L253 (-45.9117, -12.6375) -> (-46.6772, -12.6375)
  line L254 (-46.6772, -12.6375) -> (-47.9, -10.4282)
  line L255 (-47.9, -10.4282) -> (-47.9, -12.6375)
  line L256 (-47.9, -12.6375) -> (-48.627, -12.6375)
  line L257 (-48.627, -12.6375) -> (-48.627, -9.4675)
  line L258 (-48.627, -9.4675) -> (-47.6508, -9.4675)
  line L259 (-47.6508, -9.4675) -> (-46.6387, -11.2837)
  line L260 (-46.6387, -11.2837) -> (-46.6387, -9.4675)
  line L261 (-46.6387, -9.4675) -> (-45.9117, -9.4675)
  line L262 (-45.9117, -9.4675) -> (-45.9117, -12.6375)
  spline S193 degree 2 poles (-43.9003, -12.6991) (-44.6144, -12.6991) (-45.4519, -11.836) (-45.4519, -11.055) knots 0 0 0 1 2 2 2
  spline S194 degree 2 poles (-45.4519, -11.055) (-45.4519, -10.3024) (-44.6118, -9.4058) (-43.8977, -9.4058) knots 0 0 0 1 2 2 2
  spline S195 degree 2 poles (-43.8977, -9.4058) (-43.7102, -9.4058) (-43.407, -9.4495) (-43.2683, -9.4855) knots 0 0 0 1 2 2 2
  spline S196 degree 2 poles (-43.2683, -9.4855) (-43.1604, -9.5189) (-42.9061, -9.6293) (-42.8265, -9.6704) knots 0 0 0 1 2 2 2
  line L263 (-42.8265, -9.6704) -> (-42.8265, -10.4257)
  line L264 (-42.8265, -10.4257) -> (-42.9061, -10.4257)
  spline S197 degree 2 poles (-42.9061, -10.4257) (-42.9652, -10.3743) (-43.1399, -10.2304) (-43.2503, -10.1636) knots 0 0 0 1 2 2 2
  spline S198 degree 2 poles (-43.2503, -10.1636) (-43.3608, -10.0943) (-43.6254, -9.9992) (-43.7718, -9.9992) knots 0 0 0 1 2 2 2
  spline S199 degree 2 poles (-43.7718, -9.9992) (-43.9439, -9.9992) (-44.2291, -10.1071) (-44.3601, -10.2433) knots 0 0 0 1 2 2 2
  spline S200 degree 2 poles (-44.3601, -10.2433) (-44.4783, -10.364) (-44.6298, -10.7776) (-44.6298, -11.0576) knots 0 0 0 1 2 2 2
  spline S201 degree 2 poles (-44.6298, -11.0576) (-44.6298, -11.353) (-44.4731, -11.7564) (-44.3447, -11.8797) knots 0 0 0 1 2 2 2
  spline S202 degree 2 poles (-44.3447, -11.8797) (-44.2214, -12.0004) (-43.9182, -12.1057) (-43.7667, -12.1057) knots 0 0 0 1 2 2 2
  spline S203 degree 2 poles (-43.7667, -12.1057) (-43.61, -12.1057) (-43.3248, -12.0004) (-43.2272, -11.9362) knots 0 0 0 1 2 2 2
  spline S204 degree 2 poles (-43.2272, -11.9362) (-43.1193, -11.872) (-42.9575, -11.7358) (-42.8984, -11.6819) knots 0 0 0 1 2 2 2
  line L265 (-42.8984, -11.6819) -> (-42.8265, -11.6819)
  line L266 (-42.8265, -11.6819) -> (-42.8265, -12.4268)
  spline S205 degree 2 poles (-42.8265, -12.4268) (-42.9138, -12.4679) (-43.1424, -12.5707) (-43.2658, -12.6067) knots 0 0 0 1 2 2 2
  spline S206 degree 2 poles (-43.2658, -12.6067) (-43.4147, -12.6529) (-43.6742, -12.6991) (-43.9003, -12.6991) knots 0 0 0 1 2 2 2
  line L267 (-49.1819, -23.0761) -> (-51.2961, -23.0761)
  line L268 (-51.2961, -23.0761) -> (-51.2961, -19.9061)
  line L269 (-51.2961, -19.9061) -> (-50.4997, -19.9061)
  line L270 (-50.4997, -19.9061) -> (-50.4997, -22.4724)
  line L271 (-50.4997, -22.4724) -> (-49.1819, -22.4724)
  line L272 (-49.1819, -22.4724) -> (-49.1819, -23.0761)
  spline S207 degree 2 poles (-45.9168, -21.4911) (-45.9168, -22.2618) (-46.7389, -23.1429) (-47.453, -23.1429) knots 0 0 0 1 2 2 2
  spline S208 degree 2 poles (-47.453, -23.1429) (-48.1697, -23.1429) (-48.9867, -22.2515) (-48.9867, -21.4911) knots 0 0 0 1 2 2 2
  spline S209 degree 2 poles (-48.9867, -21.4911) (-48.9867, -20.7282) (-48.1697, -19.8393) (-47.453, -19.8393) knots 0 0 0 1 2 2 2
  spline S210 degree 2 poles (-47.453, -19.8393) (-46.7389, -19.8393) (-45.9168, -20.723) (-45.9168, -21.4911) knots 0 0 0 1 2 2 2
  spline S211 degree 2 poles (-46.7389, -21.4911) (-46.7389, -21.206) (-46.8545, -20.8078) (-46.9547, -20.6819) knots 0 0 0 1 2 2 2
  spline S212 degree 2 poles (-46.9547, -20.6819) (-47.0549, -20.5509) (-47.3117, -20.4379) (-47.4505, -20.4379) knots 0 0 0 1 2 2 2
  spline S213 degree 2 poles (-47.4505, -20.4379) (-47.5969, -20.4379) (-47.8358, -20.5432) (-47.9463, -20.6768) knots 0 0 0 1 2 2 2
  spline S214 degree 2 poles (-47.9463, -20.6768) (-48.0439, -20.8001) (-48.1646, -21.2085) (-48.1646, -21.4911) knots 0 0 0 1 2 2 2
  spline S215 degree 2 poles (-48.1646, -21.4911) (-48.1646, -21.784) (-48.049, -22.1693) (-47.9488, -22.3003) knots 0 0 0 1 2 2 2
  spline S216 degree 2 poles (-47.9488, -22.3003) (-47.8486, -22.4313) (-47.5892, -22.5444) (-47.4505, -22.5444) knots 0 0 0 1 2 2 2
  spline S217 degree 2 poles (-47.4505, -22.5444) (-47.3092, -22.5444) (-47.0471, -22.4236) (-46.9521, -22.2952) knots 0 0 0 1 2 2 2
  spline S218 degree 2 poles (-46.9521, -22.2952) (-46.8493, -22.1565) (-46.7389, -21.7891) (-46.7389, -21.4911) knots 0 0 0 1 2 2 2
  spline S219 degree 2 poles (-42.7982, -22.8963) (-43.0063, -22.9811) (-43.6716, -23.1429) (-43.9953, -23.1429) knots 0 0 0 1 2 2 2
  spline S220 degree 2 poles (-43.9953, -23.1429) (-44.7429, -23.1429) (-45.6291, -22.2798) (-45.6291, -21.4886) knots 0 0 0 1 2 2 2
  spline S221 degree 2 poles (-45.6291, -21.4886) (-45.6291, -20.7436) (-44.7429, -19.8445) (-43.9722, -19.8445) knots 0 0 0 1 2 2 2
  spline S222 degree 2 poles (-43.9722, -19.8445) (-43.574, -19.8445) (-43.0757, -19.996) (-42.8111, -20.1245) knots 0 0 0 1 2 2 2
  line L273 (-42.8111, -20.1245) -> (-42.8111, -20.8695)
  line L274 (-42.8111, -20.8695) -> (-42.883, -20.8695)
  spline S223 degree 2 poles (-42.883, -20.8695) (-42.9395, -20.8258) (-43.1553, -20.6588) (-43.258, -20.6023) knots 0 0 0 1 2 2 2
  spline S224 degree 2 poles (-43.258, -20.6023) (-43.3762, -20.5329) (-43.6896, -20.4353) (-43.8643, -20.4353) knots 0 0 0 1 2 2 2
  spline S225 degree 2 poles (-43.8643, -20.4353) (-44.0672, -20.4353) (-44.4038, -20.5638) (-44.5348, -20.6948) knots 0 0 0 1 2 2 2
  spline S226 degree 2 poles (-44.5348, -20.6948) (-44.6607, -20.8232) (-44.8071, -21.2163) (-44.8071, -21.4757) knots 0 0 0 1 2 2 2
  spline S227 degree 2 poles (-44.8071, -21.4757) (-44.8071, -22.0306) (-44.2496, -22.5598) (-43.7693, -22.5598) knots 0 0 0 1 2 2 2
  spline S228 degree 2 poles (-43.7693, -22.5598) (-43.7256, -22.5598) (-43.6126, -22.5546) (-43.5689, -22.5521) knots 0 0 0 1 2 2 2
  line L275 (-43.5689, -22.5521) -> (-43.5689, -21.9278)
  line L276 (-43.5689, -21.9278) -> (-44.1828, -21.9278)
  line L277 (-44.1828, -21.9278) -> (-44.1828, -21.3344)
  line L278 (-44.1828, -21.3344) -> (-42.7982, -21.3344)
  line L279 (-42.7982, -21.3344) -> (-42.7982, -22.8963)